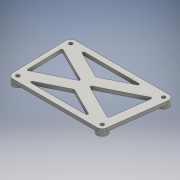
# Autodesk Inventor part: RampsMount
Saved by Autodesk Inventor 2016 (Build 200138000, 138)
## iProperties
Created: 2016-02-18
Part Number: RampsMount
Material: Generic
Document SubType Name: Modeling
Designer: Mathias L. Kjeldgaard
Density: 1 g/cm^3
Appearance: Default
Author: Mathias L. Kjeldgaard
Autodesk Inventor part; units mm, degrees
ref_plane "YZ Plane" through (0, 0, 0) normal (1, 0, 0) x (0, 1, 0)
ref_plane "XZ Plane" through (0, 0, 0) normal (0, 1, 0) x (-1, 0, 0)
ref_plane "XY Plane" through (0, 0, 0) normal (0, 0, 1) x (1, 0, 0)
sketch "Sketch1" plane through (0, 0, 0) normal (0, 0, 1) x (1, 0, 0)
  circle A0 centre (-36.83, 24.0665) radius 1.5875 projected
  circle A1 centre (45.72, 24.0665) radius 1.5875 projected
  circle A2 centre (39.37, -24.1935) radius 1.5875 projected
  circle A3 centre (-35.56, -24.1935) radius 1.5875 projected
  arc A4 (-36.83, 28.654) -> (-41.4159, 23.9458) centre (-36.83, 24.0665) ccw
  arc A5 (-40.1459, -24.3142) -> (-35.56, -28.781) centre (-35.56, -24.1935) ccw
  arc A6 (39.37, -28.781) -> (43.9183, -24.792) centre (39.37, -24.1935) ccw
  arc A7 (50.2683, 23.468) -> (45.72, 28.654) centre (45.72, 24.0665) ccw
  line L0 (50.2683, 23.468) -> (43.9183, -24.792)
  line L1 (39.37, -28.781) -> (-35.56, -28.781)
  line L2 (-40.1459, -24.3142) -> (-41.4159, 23.9458)
  line L3 (-36.83, 28.654) -> (45.72, 28.654)
  point P0 (0, 0)
  dimension "d0" = 3
  dimension "d1" = 3
  dimension "d2" = 3
  dimension "d3" = 3
  constraints: 8 end point, 8 point on circle, 8 tangent, 4 centre point
  measures "d0" radial gap between concentric circles of A0 A4
  measures "d1" radial gap between concentric circles of A3 A5
  measures "d2" radial gap between concentric circles of A2 A6
  measures "d3" radial gap between concentric circles of A1 A7
extrude "Main body" add sketch "Sketch1" along normal blind 3
sketch "Sketch3" plane through (0, 0, 0) normal (0, 0, -1) x (-1, 0, 0)
  circle A0 centre (35.56, -24.1935) radius 1.5875 projected
  circle A1 centre (-39.37, -24.1935) radius 1.5875 projected
  circle A2 centre (-45.72, 24.0665) radius 1.5875 projected
  circle A3 centre (36.83, 24.0665) radius 1.5875 projected
  circle A4 centre (35.56, -24.1935) radius 4.5875
  circle A5 centre (-39.37, -24.1935) radius 4.5875
  circle A6 centre (-45.72, 24.0665) radius 4.5875
  circle A7 centre (36.83, 24.0665) radius 4.5875
  point P0 (0, 0)
  dimension "d7" = 3
  dimension "d8" = 3
  dimension "d9" = 3
  dimension "d10" = 3
  constraints: 4 centre point
  measures "d7" radial gap between concentric circles of A0 A4
  measures "d8" radial gap between concentric circles of A3 A7
  measures "d9" radial gap between concentric circles of A2 A6
  measures "d10" radial gap between concentric circles of A1 A5
extrude "Standoff" add sketch "Sketch3" along normal blind 3
sketch "Sketch4" plane through (0, 0, 0) normal (0, 0, -1) x (-1, 0, 0)
  line L0 (28.3461, 23.654) -> (-28.3461, 23.654)
  line L1 (-28.3461, 23.654) -> (0, 9.4725)
  line L2 (0, 9.4725) -> (28.3461, 23.654)
  line L3 (37.0154, 16.8096) -> (3.4163, 0)
  line L4 (3.4163, 0) -> (36.1422, -16.3727)
  line L5 (36.1422, -16.3727) -> (37.0154, 16.8096)
  line L6 (28.5999, -23.781) -> (0, -9.4725)
  line L7 (0, -9.4725) -> (-28.5999, -23.781)
  line L8 (-28.5999, -23.781) -> (28.5999, -23.781)
  line L9 (35.56, -28.781) -> (-39.37, -28.781) projected
  line L10 (-45.72, 28.654) -> (36.83, 28.654) projected
  line L11 (-3.4163, 0) -> (-41.6219, 19.1142)
  line L12 (-41.6219, 19.1142) -> (-36.9025, -16.7531)
  line L13 (-36.9025, -16.7531) -> (-3.4163, 0)
  line L14 (-3.4163, 0) -> (3.4163, 0) construction
  line L15 (0, -9.4725) -> (0, 9.4725) construction
  line L16 (41.4159, 23.9458) -> (40.1459, -24.3142) construction
  line L17 (-43.9183, -24.792) -> (-50.2683, 23.468) construction
  point P0 (0, 0)
  dimension "d13" = 5
  dimension "d14" = 5
  dimension "d15" = 10
  dimension "d16" = 10
  dimension "d17" = 10
  dimension "d18" = 10
  constraints: 28 end point, 8 parallel, 3 horizontal, 2 midpoint, 1 vertical
  measures "d13" distance between parallel lines of L9 L8
  measures "d14" distance between parallel lines of L10 L0
  measures "d15" distance between parallel lines of L4 L6
  measures "d16" distance between parallel lines of L2 L3
  measures "d17" distance between parallel lines of L11 L1
  measures "d18" distance between parallel lines of L7 L13
extrude "Extrusion3" cut sketch "Sketch4" against normal up to surface (3 mm away)
fillet "Fillet1" radius 1 8 edges at (-28.3461, 23.654, 1.5) (28.3461, 23.654, 1.5) (41.6219, 19.1142, 1.5) (36.9025, -16.7531, 1.5) (-28.5999, -23.781, 1.5) (-36.1422, -16.3727, 1.5) (-37.0154, 16.8096, 1.5) (28.5999, -23.781, 1.5)
fillet "Fillet2" radius 2 2 edges at (0, -9.4725, 1.5) (0, 9.4725, 1.5)
fillet "Fillet3" radius 1 2 edges at (-3.4163, 0, 1.5) (3.4163, 0, 1.5)
equation "\"d1\" = d0"
equation "\"d2\" = d0"
equation "\"d3\" = d0"
equation "\"d8\" = d7"
equation "\"d9\" = d7"
equation "\"d10\" = d7"
equation "\"d14\" = d13"
equation "\"d16\" = d15"
equation "\"d17\" = d15"
equation "\"d18\" = d15"
body "Solid1"
